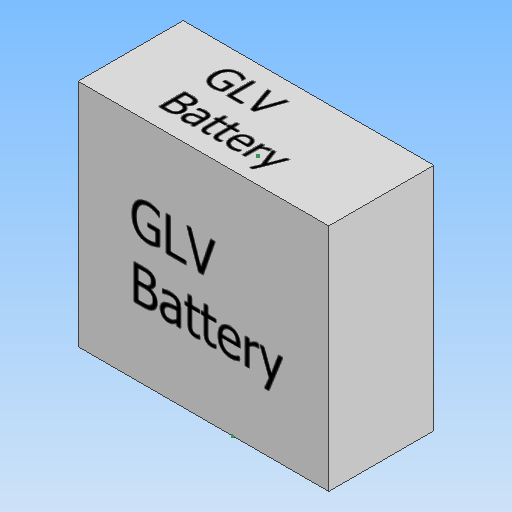
# Autodesk Inventor part: GLVBattery
Saved by Autodesk Inventor 2021 (Build 250183000, 183)
## iProperties
Created: 2020-09-13
Part Number: GLVBattery
Material: Generic
Document SubType Name: Modeling
Designer: PhotonUser
Density: 1 g/cm^3
Appearance: Default
Author: PhotonUser
Autodesk Inventor part; units mm, degrees
ref_plane "YZ Plane" through (0, 0, 0) normal (1, 0, 0) x (0, 1, 0)
ref_plane "XZ Plane" through (0, 0, 0) normal (0, 1, 0) x (-1, 0, 0)
ref_plane "XY Plane" through (0, 0, 0) normal (0, 0, 1) x (1, 0, 0)
sketch "Sketch1" plane through (0, 0, 0) normal (0, 1, 0) x (-1, 0, 0)
  line L0 (112.201, 18.1246) -> (-68.901, 18.1246)
  line L1 (-68.901, 18.1246) -> (-68.901, -57.8214)
  line L2 (-68.901, -57.8214) -> (112.201, -57.8214)
  line L3 (112.201, -57.8214) -> (112.201, 18.1246)
  point P0 (0, 0)
  dimension "d1" = 75.946
  dimension "d2" = 181.102
  constraints: 8 end point, 2 parallel, 1 horizontal, 1 perpendicular
  measures "d1" distance of L2.end L0.start
  measures "d2" distance of L0.start L0.end
extrude "Extrusion1" add sketch "Sketch1" along normal blind 166.116
sketch "Sketch2" plane through (-112.201, 0, 18.1246) normal (0, 0, 1) x (1, 0, 0)
  line L0 (37.6027, 115.8938) -> (148.168, 115.8938) construction
  line L1 (148.168, 115.8938) -> (148.168, 46.6239) construction
  line L2 (148.168, 46.6239) -> (37.6027, 46.6239) construction
  line L3 (37.6027, 46.6239) -> (37.6027, 115.8938) construction
  point P0 (112.201, 0)
  constraints: 2 other
sketch "Sketch3" plane through (0, 166.116, 0) normal (0, 1, 0) x (1, 0, 0)
  line L0 (-69.2699, 45.7359) -> (2.6642, 45.7359) construction
  line L1 (2.6642, 45.7359) -> (2.6642, 11.989) construction
  line L2 (2.6642, 11.989) -> (-69.2699, 11.989) construction
  line L3 (-69.2699, 11.989) -> (-69.2699, 45.7359) construction
  point P0 (0, 0)
  constraints: 2 other
equation "\"d1\" = BatteryWidth"
equation "\"d2\" = BatteryLength"
equation "\"d3\" = BatteryHeight"
equation "\"BatteryLength\" = 181.102"
equation "\"BatteryWidth\" = 75.946"
equation "\"BatteryHeight\" = 166.116"
body "Solid1"
